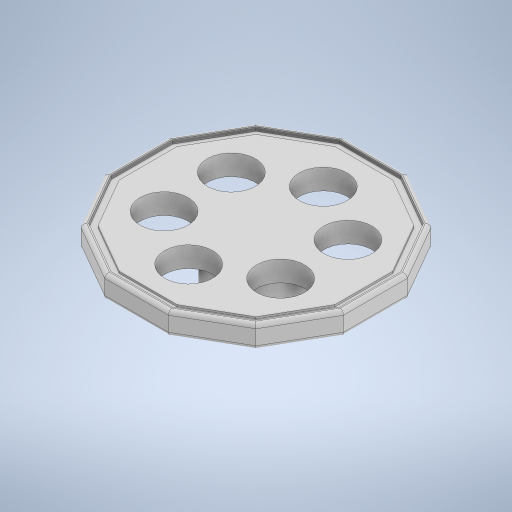
# Autodesk Inventor part: OV-PAM_n_12_bottom
Saved by Autodesk Inventor 2024 (Build 280153000, 153)
## iProperties
Created: 2023-08-31
Part Number: OV-PAM_n_12_bottom
Material: 일반
Document SubType Name: Modeling
Designer: jsw
Density: 1 g/cm^3
Appearance: 기본값
Author: jsw
Autodesk Inventor part; units mm, degrees
ref_plane "YZ Plane" through (0, 0, 0) normal (1, 0, 0) x (0, 1, 0)
ref_plane "XZ Plane" through (0, 0, 0) normal (0, 1, 0) x (-1, 0, 0)
ref_plane "XY Plane" through (0, 0, 0) normal (0, 0, 1) x (1, 0, 0)
sketch "스케치1" plane through (0, 0, 0) normal (0, 1, 0) x (-1, 0, 0)
  line L0 (24.9446, -24.9446) -> (9.1304, -34.075)
  line L1 (9.1304, -34.075) -> (-9.1304, -34.075)
  line L2 (-9.1304, -34.075) -> (-24.9446, -24.9446)
  line L3 (-24.9446, -24.9446) -> (-34.075, -9.1304)
  line L4 (-34.075, -9.1304) -> (-34.075, 9.1304)
  line L5 (-34.075, 9.1304) -> (-24.9446, 24.9446)
  line L6 (-24.9446, 24.9446) -> (-9.1304, 34.075)
  line L7 (-9.1304, 34.075) -> (9.1304, 34.075)
  line L8 (9.1304, 34.075) -> (24.9446, 24.9446)
  line L9 (24.9446, 24.9446) -> (34.075, 9.1304)
  line L10 (34.075, 9.1304) -> (34.075, -9.1304)
  line L11 (34.075, -9.1304) -> (24.9446, -24.9446)
  line L12 (9.9878, -37.275) -> (-9.9878, -37.275)
  line L13 (-9.9878, -37.275) -> (-27.2872, -27.2872)
  line L14 (-27.2872, -27.2872) -> (-37.275, -9.9878)
  line L15 (-37.275, -9.9878) -> (-37.275, 9.9878)
  line L16 (-37.275, 9.9878) -> (-27.2872, 27.2872)
  line L17 (-27.2872, 27.2872) -> (-9.9878, 37.275)
  line L18 (-9.9878, 37.275) -> (9.9878, 37.275)
  line L19 (9.9878, 37.275) -> (27.2872, 27.2872)
  line L20 (27.2872, 27.2872) -> (37.275, 9.9878)
  line L21 (37.275, 9.9878) -> (37.275, -9.9878)
  line L22 (37.275, -9.9878) -> (27.2872, -27.2872)
  line L23 (27.2872, -27.2872) -> (9.9878, -37.275)
  point P0 (0, 0)
  point P1 (0, 0)
  point P2 (0, 0)
  dimension "d0" = 70.554
  dimension "d1" = 3.2
  constraints: 48 end point, 2 coincident, 2 horizontal, 50 other
  measures "d0" distance of L3.end L9.end
  measures "d1" distance between parallel lines of L10 L21
extrude "돌출1" add sketch "스케치1" along normal blind 7 contours L0 L1 L2 L3 L4 L5 L6 L7 L8 L9 L10 L11 | L12 L13 L14 L15 L16 L17 L18 L19 L20 L21 L22 L23
sketch "스케치2" plane through (0, 7, 0) normal (0, 1, 0) x (1, 0, 0)
  line L0 (-9.5591, 35.675) -> (9.5591, 35.675)
  line L1 (9.5591, 35.675) -> (26.1159, 26.1159)
  line L2 (26.1159, 26.1159) -> (35.675, 9.5591)
  line L3 (35.675, 9.5591) -> (35.675, -9.5591)
  line L4 (35.675, -9.5591) -> (26.1159, -26.1159)
  line L5 (26.1159, -26.1159) -> (9.5591, -35.675)
  line L6 (9.5591, -35.675) -> (-9.5591, -35.675)
  line L7 (-9.5591, -35.675) -> (-26.1159, -26.1159)
  line L8 (-26.1159, -26.1159) -> (-35.675, -9.5591)
  line L9 (-35.675, -9.5591) -> (-35.675, 9.5591)
  line L10 (-35.675, 9.5591) -> (-26.1159, 26.1159)
  line L11 (-26.1159, 26.1159) -> (-9.5591, 35.675)
  line L12 (9.9878, 37.275) -> (-9.9878, 37.275) projected
  point P0 (0, 0)
  point P1 (0, 0)
  point P2 (0, 35.675)
  dimension "d4" = 1.6
  constraints: 24 end point, 1 coincident, 1 horizontal, 1 midpoint, 25 other
  measures "d4" distance from line of L12 point (0, 35.675)
extrude "돌출2" cut sketch "스케치2" against normal blind 1.2
sketch "스케치3" plane through (0, 5.8, 0) normal (0, 1, 0) x (1, 0, 0)
  line L0 (-9.0232, 33.675) -> (9.0232, 33.675)
  line L1 (9.0232, 33.675) -> (24.6518, 24.6518)
  line L2 (24.6518, 24.6518) -> (33.675, 9.0232)
  line L3 (33.675, 9.0232) -> (33.675, -9.0232)
  line L4 (33.675, -9.0232) -> (24.6518, -24.6518)
  line L5 (24.6518, -24.6518) -> (9.0232, -33.675)
  line L6 (9.0232, -33.675) -> (-9.0232, -33.675)
  line L7 (-9.0232, -33.675) -> (-24.6518, -24.6518)
  line L8 (-24.6518, -24.6518) -> (-33.675, -9.0232)
  line L9 (-33.675, -9.0232) -> (-33.675, 9.0232)
  line L10 (-33.675, 9.0232) -> (-24.6518, 24.6518)
  line L11 (-24.6518, 24.6518) -> (-9.0232, 33.675)
  line L12 (-9.5591, 35.675) -> (9.5591, 35.675) projected
  point P0 (0, 0)
  point P1 (0, 0)
  dimension "d7" = 2
  constraints: 24 end point, 1 coincident, 1 horizontal, 25 other
  measures "d7" distance between parallel lines of L12 L0
extrude "돌출3" add sketch "스케치3" along normal blind 0.6
fillet "모깎기1" radius 1.2 24 edges at (-18.6375, 7, 32.2811) (-32.2811, 7, 18.6375) (-37.275, 7, 0) (0, 7, 37.275) (18.6375, 7, 32.2811) (32.2811, 7, 18.6375) (37.275, 7, 0) (32.2811, 7, -18.6375) (18.6375, 7, -32.2811) (0, 7, -37.275) (-18.6375, 7, -32.2811) (-32.2811, 7, -18.6375) (-37.275, 0, 0) (-32.2811, 0, 18.6375) (-18.6375, 0, 32.2811) (0, 0, 37.275) (18.6375, 0, 32.2811) (32.2811, 0, 18.6375) (37.275, 0, 0) (32.2811, 0, -18.6375) (18.6375, 0, -32.2811) (0, 0, -37.275) (-18.6375, 0, -32.2811) (-32.2811, 0, -18.6375)
sketch "스케치11" plane through (0, 0, 0) normal (0, -1, 0) x (1, 0, 0)
  circle A0 centre (0, 0) radius 12.7
  dimension "d48" = 25.4
  constraints: 1 centre point, 1 coincident
  measures "d48" diameter of A0
extrude "돌출11" add sketch "스케치11" along normal blind 10.16
sketch "스케치12" plane through (0, -10.16, 0) normal (0, -1, 0) x (1, 0, 0)
  circle A0 centre (0, 0) radius 3.9688
  dimension "d51" = 7.9375
  constraints: 1 centre point, 1 coincident
  measures "d51" diameter of A0
extrude "돌출12" cut sketch "스케치12" against normal blind 10.16
thread "스레드1" size "5/16-18 UNC" class "2B" standard "ANSI Unified Screw Threads" full length
sketch "스케치13" plane through (0, 0, 0) normal (0, -1, 0) x (1, 0, 0)
  circle A0 centre (0, -21) radius 7.5
  circle A1 centre (18.1865, -10.5) radius 7.5
  circle A2 centre (18.1865, 10.5) radius 7.5
  circle A3 centre (0, 21) radius 7.5
  circle A4 centre (-18.1865, 10.5) radius 7.5
  circle A5 centre (-18.1865, -10.5) radius 7.5
  point P0 (0, 0)
  dimension "d56" = 15
  dimension "d57" = 21
  dimension "d60" = 360
  constraints: 6 centre point, 1 vertical alignment, 13 other
  measures "d56" diameter of A0
  measures "d57" distance of A0.centre point (0, 0)
extrude "돌출13" cut sketch "스케치13" against normal up to surface (6.4 mm away)
sketch "스케치15" plane through (0, 0, 0) normal (1, 0, 0) x (0, 0, 1)
  line L0 (3.9688, 0) -> (3.9688, 10.16)
  line L1 (3.9688, 10.16) -> (2.9225, 10.16)
  line L2 (2.9225, 10.16) -> (2.9225, 0)
  line L3 (2.9225, 0) -> (3.9688, 0)
  line L4 (0, -10.432) -> (0, 13.592) projected
  constraints: 8 end point
revolve "회전1" add sketch "스케치15" angle 360 about axis through (0, 0, 0) along (0, -1, 0) separate body
sketch "스케치14" plane through (0, 0, 3.9688) normal (-1, 0, 0) x (0, -1, 0)
  line L0 (-0.8233, -0.0715) -> (-0.7057, -0.0715) construction
  line L1 (0.1175, -0.9751) -> (-0.0001, -1.201) construction
  line L2 (-1.4112, -1.201) -> (-1.5288, -0.9751) construction
  line L3 (-0.5881, -0.0715) -> (-0.7057, 0.1544) construction
  line L4 (-0.7057, 0.1544) -> (-0.8233, -0.0715) construction
  line L5 (-1.4112, -1.201) -> (-1.2936, -0.9751) construction
  line L6 (-0.5881, -0.0715) -> (-0.1177, -0.9751)
  line L7 (-1.5288, -0.9751) -> (-1.2936, -0.9751) construction
  arc A0 (-1.5288, -0.9751) -> (-1.4112, -1.0465) centre (-1.4112, -0.9139) ccw construction
  line L8 (0.1175, -0.9751) -> (-0.1177, -0.9751) construction
  line L9 (-1.4112, -1.201) -> (-1.4112, -0.9751) construction
  line L10 (-0.0001, -1.201) -> (-0.0001, -0.9751) construction
  line L11 (-0.7057, 0.1544) -> (-0.7057, -0.0002) construction
  line L12 (-1.4112, -1.0465) -> (-0.0001, -1.0465)
  arc A1 (-1.4112, -1.0465) -> (-1.2936, -0.9751) centre (-1.4112, -0.9139) ccw
  line L13 (-0.1177, -0.9751) -> (-0.0001, -1.201) construction
  line L14 (-1.2936, -0.9751) -> (-0.8233, -0.0715)
  line L15 (-0.0001, -0.0002) -> (-0.0001, 0.0177)
  line L16 (-0.0001, 0.0177) -> (-0.0001, -0.0002)
  line L17 (-0.0001, -0.0002) -> (0.0334, -0.0002)
  arc A2 (-0.1177, -0.9751) -> (-0.0001, -1.0465) centre (-0.0001, -0.9139) ccw
  arc A3 (-0.0001, -1.0465) -> (0.1175, -0.9751) centre (-0.0001, -0.9139) ccw construction
  arc A4 (-0.7057, -0.0002) -> (-0.8233, -0.0715) centre (-0.7057, -0.1327) ccw
  arc A5 (-0.5881, -0.0715) -> (-0.7057, -0.0002) centre (-0.7057, -0.1327) ccw
  line L18 (-0.7057, -0.0002) -> (-0.7057, -0.0715) construction
  line L19 (-0.7057, -0.0715) -> (-0.5881, -0.0715) construction
  dimension "d64" = 55
  dimension "d65" = 0.2259
  dimension "d66" = 0.2259
  dimension "d69" = 1.4111
  constraints: 40 end point, 12 point on circle, 10 parallel, 9 tangent, 7 collinear, 6 centre point, 2 midpoint, 2 point on line, 1 horizontal, 1 perpendicular, 4 other
  measures "d64" angle of L6 L14
  measures "d65" distance of L3.end L0.end
  measures "d66" distance of L1.end L10.end
  measures "d69" distance from line of L1.end L9
coil "코일1" sketch "스케치14" operation cut axis through (0, 0, 0) along (0, -1, 0) pitch 1.4125 turns 9.190809 hand right bodies 2
equation "\"d64\" = d71"
equation "\"d71\" = 55deg"
